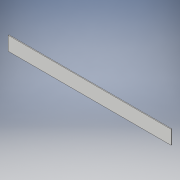
# Autodesk Inventor part: plastic wall
Saved by Autodesk Inventor 2019 (Build 230136000, 136)
## iProperties
Created: 2021-07-19
Part Number: plastic wall
Material: Generic
Document SubType Name: Modeling
Designer: pensun
Density: 1 g/cm^3
Appearance: Default
Author: pensun
Autodesk Inventor part; units mm, degrees
ref_plane "YZ Plane" through (0, 0, 0) normal (1, 0, 0) x (0, 1, 0)
ref_plane "XZ Plane" through (0, 0, 0) normal (0, 1, 0) x (-1, 0, 0)
ref_plane "XY Plane" through (0, 0, 0) normal (0, 0, 1) x (1, 0, 0)
sketch "Sketch1" plane through (0, 0, 0) normal (0, 0, 1) x (1, 0, 0)
  line L0 (-500, 42.5) -> (500, 42.5)
  line L1 (500, 42.5) -> (500, -42.5)
  line L2 (500, -42.5) -> (-500, -42.5)
  line L3 (-500, -42.5) -> (-500, 42.5)
  point P0 (0, 0)
  dimension "d0" = 42.5
  dimension "d1" = 1000
  dimension "d2" = 85
  dimension "d3" = 500
  constraints: 8 end point, 2 parallel, 1 horizontal, 1 perpendicular
  measures "d0" distance from line of point (0, 0) L0
  measures "d1" distance of L0.start L0.end
  measures "d2" distance of L0.end L1.end
  measures "d3" distance from line of L3 point (0, 0)
extrude "Extrusion1" add sketch "Sketch1" along normal blind 5
equation "\"d0\" = 0.5 * d2"
equation "\"d3\" = 0.5 * d1"
body "Solid1"
